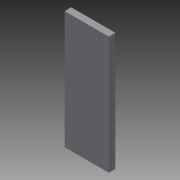
# Autodesk Inventor part: Base
Saved by Autodesk Inventor 2014 (Build 180170000, 170)
## iProperties
Created: 2016-02-02
Part Number: Base
Material: Generic
Document SubType Name: Modeling
Designer: sametj
Density: 1 g/cm^3
Appearance: Default
Author: sametj
Autodesk Inventor part; units mm, degrees
ref_plane "YZ Plane" through (0, 0, 0) normal (1, 0, 0) x (0, 1, 0)
ref_plane "XZ Plane" through (0, 0, 0) normal (0, 1, 0) x (-1, 0, 0)
ref_plane "XY Plane" through (0, 0, 0) normal (0, 0, 1) x (1, 0, 0)
sketch "Sketch1" plane through (0, 0, 0) normal (0, 0, 1) x (1, 0, 0)
  line L0 (-104.9821, 95.3535) -> (-19.2571, 95.3535)
  line L1 (-19.2571, 95.3535) -> (-19.2571, -133.2465)
  line L2 (-19.2571, -133.2465) -> (-104.9821, -133.2465)
  line L3 (-104.9821, -133.2465) -> (-104.9821, 95.3535)
  point P0 (0, 0)
  dimension "d0" = 228.6
  dimension "d1" = 85.725
  constraints: 8 end point, 2 parallel, 1 horizontal, 1 perpendicular
  measures "d0" distance of L2.end L0.start
  measures "d1" distance of L0.start L0.end
extrude "Extrusion1" add sketch "Sketch1" along normal blind 12.7
body "Solid1"
